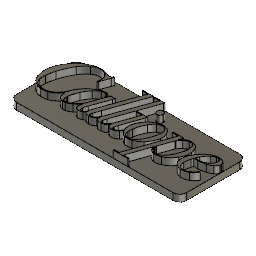
Calliope_Logo (Autodesk Fusion 360 design; units mm, degrees)
Autodesk Fusion 360 part; units mm, degrees
note: some values were not read from the file. Chosen so that the rebuilt part matches the saved one: which pieces of a blend or face edit are solid. Set by a fixed rule: which sketch regions a step uses.
(part 1 of 3)
sketch "Sketch3" plane through (0, 0, 0) normal (0, 0, 1) x (1, 0, 0)
  line L0 (156.0195, -23.5976) -> (156.0195, -61.341)
  line L1 (156.0195, -61.341) -> (108.4773, -61.341)
  spline S0 degree 3 poles (108.4773, -61.341) (108.5491, -61.0596) (108.6209, -60.7783) (108.7043, -60.4516) knots 0 0 0 0 1 1 1 1
  line L2 (108.7043, -60.4516) -> (103.7692, -60.4516)
  spline S1 degree 3 poles (103.7692, -60.4516) (106.1753, -53.6131) (108.5658, -46.8189) (110.9796, -39.9584) knots 0 0 0 0 1 1 1 1
  spline S2 degree 3 poles (110.9796, -39.9584) (111.1778, -40.6135) (111.3001, -41.1945) (111.5257, -41.7321) knots 0 0 0 0 1 1 1 1
  spline S3 degree 3 poles (111.5257, -41.7321) (112.4488, -43.9326) (114.0522, -45.3171) (116.4762, -45.532) knots 0 0 0 0 1 1 1 1
  spline S4 degree 3 poles (116.4762, -45.532) (118.5105, -45.7123) (120.4877, -45.3426) (122.343, -44.485) knots 0 0 0 0 1 1 1 1
  spline S5 degree 3 poles (122.343, -44.485) (125.9058, -42.8382) (128.6456, -40.264) (130.6312, -36.8985) knots 0 0 0 0 1 1 1 1
  spline S6 degree 3 poles (130.6312, -36.8985) (132.3382, -34.0054) (133.3231, -30.9198) (132.9158, -27.5036) knots 0 0 0 0 1 1 1 1
  spline S7 degree 3 poles (132.9158, -27.5036) (132.7164, -25.831) (132.2982, -24.2283) (131.4403, -22.7614) knots 0 0 0 0 1 1 1 1
  spline S8 degree 3 poles (131.4403, -22.7614) (129.2488, -19.0142) (125.0975, -18.1221) (121.9017, -19.2309) knots 0 0 0 0 1 1 1 1
  spline S9 degree 3 poles (121.9017, -19.2309) (119.7817, -19.9664) (118.1223, -21.3511) (116.8137, -23.1628) knots 0 0 0 0 1 1 1 1
  spline S10 degree 3 poles (116.8137, -23.1628) (116.7552, -23.2438) (116.6934, -23.3224) (116.6331, -23.4021) knots 0 0 0 0 1 1 1 1
  line L3 (116.6331, -23.4021) -> (116.5718, -23.3725)
  spline S11 degree 3 poles (116.5718, -23.3725) (116.9751, -22.1176) (117.3783, -20.8626) (117.794, -19.5691) knots 0 0 0 0 1 1 1 1
  line L4 (117.794, -19.5691) -> (117.39, -19.5691)
  spline S12 degree 3 poles (117.39, -19.5691) (116.1524, -19.5691) (114.9147, -19.5691) (113.677, -19.5691) knots 0 0 0 0 1 1 1 1
  spline S13 degree 3 poles (113.677, -19.5691) (112.0374, -19.5691) (110.3977, -19.567) (108.7581, -19.5739) knots 0 0 0 0 1 1 1 1
  spline S14 degree 3 poles (108.7581, -19.5739) (108.6477, -19.5743) (108.4711, -19.6131) (108.4397, -19.6844) knots 0 0 0 0 1 1 1 1
  spline S15 degree 3 poles (108.4397, -19.6844) (108.3413, -19.9076) (108.2979, -20.1549) (108.2252, -20.4221) knots 0 0 0 0 1 1 1 1
  line L5 (108.2252, -20.4221) -> (113.6878, -20.4221)
  spline S16 degree 3 poles (113.6878, -20.4221) (113.6473, -20.5473) (113.6177, -20.6465) (113.5834, -20.7441) knots 0 0 0 0 1 1 1 1
  spline S17 degree 3 poles (113.5834, -20.7441) (108.9605, -33.8922) (104.3365, -47.04) (99.7194, -60.1902) knots 0 0 0 0 1 1 1 1
  spline S18 degree 3 poles (99.7194, -60.1902) (99.6414, -60.4125) (99.533, -60.4699) (99.3115, -60.4681) knots 0 0 0 0 1 1 1 1
  spline S19 degree 3 poles (99.3115, -60.4681) (98.0845, -60.4581) (96.8573, -60.46) (95.6303, -60.4696) knots 0 0 0 0 1 1 1 1
  spline S20 degree 3 poles (95.6303, -60.4696) (95.5302, -60.4704) (95.3717, -60.5363) (95.342, -60.6118) knots 0 0 0 0 1 1 1 1
  spline S21 degree 3 poles (95.342, -60.6118) (95.2508, -60.8445) (95.2089, -61.0965) (95.1478, -61.341) knots 0 0 0 0 1 1 1 1
  line L6 (95.1478, -61.341) -> (0, -61.341)
  line L7 (0, -61.341) -> (0, 0)
  spline S22 degree 3 poles (0, 0) (52.0065, 0) (104.013, 0) (156.0195, 0) knots 0 0 0 0 1 1 1 1
  line L8 (156.0195, 0) -> (156.0195, -22.8998)
  spline S23 degree 3 poles (156.0195, -22.8998) (156.0019, -22.8646) (155.9715, -22.8305) (155.9685, -22.7942) knots 0 0 0 0 1 1 1 1
  spline S24 degree 3 poles (155.9685, -22.7942) (155.8892, -21.8192) (155.4189, -21.052) (154.6851, -20.4397) knots 0 0 0 0 1 1 1 1
  spline S25 degree 3 poles (154.6851, -20.4397) (153.4053, -19.3719) (151.8701, -18.9809) (150.2562, -18.8437) knots 0 0 0 0 1 1 1 1
  spline S26 degree 3 poles (150.2562, -18.8437) (147.8053, -18.6354) (145.5366, -19.2454) (143.4312, -20.4739) knots 0 0 0 0 1 1 1 1
  spline S27 degree 3 poles (143.4312, -20.4739) (139.1005, -23.0008) (136.0205, -26.6341) (134.0532, -31.2182) knots 0 0 0 0 1 1 1 1
  spline S28 degree 3 poles (134.0532, -31.2182) (133.1018, -33.4352) (132.6126, -35.7441) (132.9818, -38.1701) knots 0 0 0 0 1 1 1 1
  spline S29 degree 3 poles (132.9818, -38.1701) (133.2638, -40.0236) (133.9884, -41.6782) (135.3221, -43.0231) knots 0 0 0 0 1 1 1 1
  spline S30 degree 3 poles (135.3221, -43.0231) (136.8021, -44.5156) (138.6131, -45.3113) (140.7013, -45.5057) knots 0 0 0 0 1 1 1 1
  spline S31 degree 3 poles (140.7013, -45.5057) (143.1519, -45.7339) (145.4639, -45.3818) (147.6206, -44.0951) knots 0 0 0 0 1 1 1 1
  spline S32 degree 3 poles (147.6206, -44.0951) (149.696, -42.8569) (151.1962, -41.1095) (152.41, -39.0493) knots 0 0 0 0 1 1 1 1
  spline S33 degree 3 poles (152.41, -39.0493) (152.1937, -38.9254) (151.9691, -38.7968) (151.7296, -38.6596) knots 0 0 0 0 1 1 1 1
  spline S34 degree 3 poles (151.7296, -38.6596) (151.52, -38.9343) (151.3182, -39.1785) (151.1384, -39.4379) knots 0 0 0 0 1 1 1 1
  spline S35 degree 3 poles (151.1384, -39.4379) (150.286, -40.6676) (149.3449, -41.8167) (148.1741, -42.7628) knots 0 0 0 0 1 1 1 1
  spline S36 degree 3 poles (148.1741, -42.7628) (146.3193, -44.2615) (144.246, -45.0682) (141.8277, -44.718) knots 0 0 0 0 1 1 1 1
  spline S37 degree 3 poles (141.8277, -44.718) (139.955, -44.4468) (138.4938, -43.5447) (137.642, -41.8068) knots 0 0 0 0 1 1 1 1
  spline S38 degree 3 poles (137.642, -41.8068) (137.1687, -40.8411) (137.0345, -39.7935) (137.0087, -38.7285) knots 0 0 0 0 1 1 1 1
  spline S39 degree 3 poles (137.0087, -38.7285) (136.9596, -36.7106) (137.328, -34.757) (137.9094, -32.836) knots 0 0 0 0 1 1 1 1
  spline S40 degree 3 poles (137.9094, -32.836) (138.1099, -32.1735) (138.3185, -31.5134) (138.503, -30.9178) knots 0 0 0 0 1 1 1 1
  spline S41 degree 3 poles (138.503, -30.9178) (139.7894, -30.9729) (141.0146, -31.0989) (142.2347, -31.0619) knots 0 0 0 0 1 1 1 1
  spline S42 degree 3 poles (142.2347, -31.0619) (144.493, -30.9934) (146.7045, -30.5779) (148.8648, -29.9105) knots 0 0 0 0 1 1 1 1
  spline S43 degree 3 poles (148.8648, -29.9105) (150.5076, -29.403) (152.0871, -28.7496) (153.4759, -27.7167) knots 0 0 0 0 1 1 1 1
  spline S44 degree 3 poles (153.4759, -27.7167) (154.6089, -26.874) (155.5238, -25.8533) (155.8582, -24.4251) knots 0 0 0 0 1 1 1 1
  spline S45 degree 3 poles (155.8582, -24.4251) (155.9223, -24.1517) (155.9663, -23.8735) (156.0195, -23.5976) knots 0 0 0 0 1 1 1 1
  spline S46 degree 3 poles (50.0849, -22.4452) (50.0619, -22.439) (50.0388, -22.4327) (50.0158, -22.4265) knots 0 0 0 0 1 1 1 1
  spline S47 degree 3 poles (50.0158, -22.4265) (50.0064, -22.3974) (49.9927, -22.3689) (49.9884, -22.3392) knots 0 0 0 0 1 1 1 1
  spline S48 degree 3 poles (49.9884, -22.3392) (49.9779, -22.2661) (49.9693, -22.1925) (49.9641, -22.1189) knots 0 0 0 0 1 1 1 1
  spline S49 degree 3 poles (49.9641, -22.1189) (49.8984, -21.1818) (49.4912, -20.4209) (48.7702, -19.8267) knots 0 0 0 0 1 1 1 1
  spline S50 degree 3 poles (48.7702, -19.8267) (47.7681, -19.0007) (46.5961, -18.7389) (45.3289, -18.8182) knots 0 0 0 0 1 1 1 1
  spline S51 degree 3 poles (45.3289, -18.8182) (43.9034, -18.9073) (42.5718, -19.3541) (41.2975, -19.9603) knots 0 0 0 0 1 1 1 1
  spline S52 degree 3 poles (41.2975, -19.9603) (37.4617, -21.785) (34.2471, -24.4068) (31.5841, -27.6967) knots 0 0 0 0 1 1 1 1
  spline S53 degree 3 poles (31.5841, -27.6967) (29.8681, -29.8167) (28.5608, -32.172) (27.7761, -34.8009) knots 0 0 0 0 1 1 1 1
  spline S54 degree 3 poles (27.7761, -34.8009) (27.6548, -35.2071) (27.6013, -35.6146) (27.2979, -35.9909) knots 0 0 0 0 1 1 1 1
  spline S55 degree 3 poles (27.2979, -35.9909) (26.7981, -36.6105) (26.4452, -37.3469) (26.0145, -38.024) knots 0 0 0 0 1 1 1 1
  spline S56 degree 3 poles (26.0145, -38.024) (24.3785, -40.5957) (22.1935, -42.5594) (19.4153, -43.8207) knots 0 0 0 0 1 1 1 1
  spline S57 degree 3 poles (19.4153, -43.8207) (16.336, -45.2186) (13.1649, -45.1705) (10.0109, -44.1478) knots 0 0 0 0 1 1 1 1
  spline S58 degree 3 poles (10.0109, -44.1478) (7.3021, -43.2695) (5.6053, -41.3794) (4.9304, -38.5933) knots 0 0 0 0 1 1 1 1
  spline S59 degree 3 poles (4.9304, -38.5933) (4.4781, -36.726) (4.5193, -34.842) (4.7229, -32.9543) knots 0 0 0 0 1 1 1 1
  spline S60 degree 3 poles (4.7229, -32.9543) (5.0136, -30.2599) (5.5761, -27.6183) (6.3535, -25.0241) knots 0 0 0 0 1 1 1 1
  spline S61 degree 3 poles (6.3535, -25.0241) (7.7161, -20.4766) (9.4965, -16.1067) (12.0128, -12.064) knots 0 0 0 0 1 1 1 1
  spline S62 degree 3 poles (12.0128, -12.064) (13.6498, -9.4342) (15.5983, -7.0752) (18.1065, -5.2075) knots 0 0 0 0 1 1 1 1
  spline S63 degree 3 poles (18.1065, -5.2075) (21.6115, -2.5974) (25.4024, -2.3618) (29.3636, -3.8873) knots 0 0 0 0 1 1 1 1
  spline S64 degree 3 poles (29.3636, -3.8873) (31.4072, -4.6744) (32.7504, -6.1919) (33.298, -8.3429) knots 0 0 0 0 1 1 1 1
  spline S65 degree 3 poles (33.298, -8.3429) (33.6344, -9.6642) (33.5355, -11.0084) (33.4161, -12.3468) knots 0 0 0 0 1 1 1 1
  spline S66 degree 3 poles (33.4161, -12.3468) (33.3593, -12.9843) (33.2661, -13.6185) (33.1895, -14.2539) knots 0 0 0 0 1 1 1 1
  spline S67 degree 3 poles (33.1895, -14.2539) (33.924, -14.3486) (33.9218, -14.3478) (34.1497, -13.71) knots 0 0 0 0 1 1 1 1
  spline S68 degree 3 poles (34.1497, -13.71) (35.1509, -10.908) (36.1535, -8.1065) (37.1555, -5.3048) knots 0 0 0 0 1 1 1 1
  spline S69 degree 3 poles (37.1555, -5.3048) (37.4387, -4.513) (37.7215, -3.721) (38.014, -2.9026) knots 0 0 0 0 1 1 1 1
  spline S70 degree 3 poles (38.014, -2.9026) (37.8301, -2.8616) (37.6735, -2.8421) (37.5281, -2.7909) knots 0 0 0 0 1 1 1 1
  spline S71 degree 3 poles (37.5281, -2.7909) (37.2322, -2.6868) (37.0752, -2.7732) (36.9084, -3.0554) knots 0 0 0 0 1 1 1 1
  spline S72 degree 3 poles (36.9084, -3.0554) (36.3629, -3.9783) (35.5622, -4.5251) (34.4509, -4.4166) knots 0 0 0 0 1 1 1 1
  spline S73 degree 3 poles (34.4509, -4.4166) (33.9099, -4.3637) (33.3658, -4.2376) (32.8488, -4.0667) knots 0 0 0 0 1 1 1 1
  spline S74 degree 3 poles (32.8488, -4.0667) (31.9676, -3.7753) (31.1102, -3.4127) (30.2365, -3.0973) knots 0 0 0 0 1 1 1 1
  spline S75 degree 3 poles (30.2365, -3.0973) (27.7778, -2.2096) (25.2539, -1.9088) (22.6573, -2.2749) knots 0 0 0 0 1 1 1 1
  spline S76 degree 3 poles (22.6573, -2.2749) (20.7362, -2.5458) (18.9175, -3.1537) (17.1711, -3.9759) knots 0 0 0 0 1 1 1 1
  spline S77 degree 3 poles (17.1711, -3.9759) (11.8716, -6.4708) (7.6391, -10.2081) (4.4487, -15.0988) knots 0 0 0 0 1 1 1 1
  spline S78 degree 3 poles (4.4487, -15.0988) (1.4603, -19.6798) (-0.1988, -24.667) (0.1153, -30.2088) knots 0 0 0 0 1 1 1 1
  spline S79 degree 3 poles (0.1153, -30.2088) (0.2462, -32.5189) (0.589, -34.789) (1.4018, -36.9651) knots 0 0 0 0 1 1 1 1
  spline S80 degree 3 poles (1.4018, -36.9651) (2.7269, -40.5128) (5.07, -43.1219) (8.5869, -44.6156) knots 0 0 0 0 1 1 1 1
  spline S81 degree 3 poles (8.5869, -44.6156) (9.982, -45.2081) (11.4556, -45.483) (12.9615, -45.5794) knots 0 0 0 0 1 1 1 1
  spline S82 degree 3 poles (12.9615, -45.5794) (14.9147, -45.7043) (16.8656, -45.6654) (18.7272, -44.9928) knots 0 0 0 0 1 1 1 1
  spline S83 degree 3 poles (18.7272, -44.9928) (22.1612, -43.7524) (24.8613, -41.5667) (26.8476, -38.5034) knots 0 0 0 0 1 1 1 1
  spline S84 degree 3 poles (26.8476, -38.5034) (26.988, -38.287) (27.118, -38.0638) (27.2529, -37.8437) knots 0 0 0 0 1 1 1 1
  spline S85 degree 3 poles (27.2529, -37.8437) (27.3252, -37.9926) (27.3127, -38.1253) (27.3273, -38.2549) knots 0 0 0 0 1 1 1 1
  spline S86 degree 3 poles (27.3273, -38.2549) (27.4213, -39.0926) (27.4431, -39.948) (27.6348, -40.7633) knots 0 0 0 0 1 1 1 1
  spline S87 degree 3 poles (27.6348, -40.7633) (28.0824, -42.6659) (29.1177, -44.1579) (30.9434, -45.0023) knots 0 0 0 0 1 1 1 1
  spline S88 degree 3 poles (30.9434, -45.0023) (32.3176, -45.6378) (33.7642, -45.6821) (35.2298, -45.4504) knots 0 0 0 0 1 1 1 1
  spline S89 degree 3 poles (35.2298, -45.4504) (37.0632, -45.1607) (38.6343, -44.293) (40.0946, -43.1941) knots 0 0 0 0 1 1 1 1
  spline S90 degree 3 poles (40.0946, -43.1941) (41.6556, -42.0196) (42.8844, -40.5225) (44.1283, -39.0402) knots 0 0 0 0 1 1 1 1
  spline S91 degree 3 poles (44.1283, -39.0402) (44.2114, -38.9412) (44.2975, -38.8447) (44.3823, -38.747) knots 0 0 0 0 1 1 1 1
  spline S92 degree 3 poles (44.3823, -38.747) (44.4123, -38.9053) (44.3802, -39.0239) (44.3478, -39.1425) knots 0 0 0 0 1 1 1 1
  spline S93 degree 3 poles (44.3478, -39.1425) (44.0412, -40.2656) (43.7805, -41.3953) (43.8608, -42.5731) knots 0 0 0 0 1 1 1 1
  spline S94 degree 3 poles (43.8608, -42.5731) (43.9596, -44.0239) (44.7538, -45.0434) (46.147, -45.3786) knots 0 0 0 0 1 1 1 1
  spline S95 degree 3 poles (46.147, -45.3786) (47.775, -45.7703) (49.3655, -45.6409) (50.8342, -44.773) knots 0 0 0 0 1 1 1 1
  spline S96 degree 3 poles (50.8342, -44.773) (51.4483, -44.4101) (52.0194, -43.9749) (52.6073, -43.5745) knots 0 0 0 0 1 1 1 1
  spline S97 degree 3 poles (52.6073, -43.5745) (53.0764, -44.5495) (53.5786, -45.0228) (54.6679, -45.2941) knots 0 0 0 0 1 1 1 1
  spline S98 degree 3 poles (54.6679, -45.2941) (55.3375, -45.4608) (56.041, -45.5543) (56.731, -45.5649) knots 0 0 0 0 1 1 1 1
  spline S99 degree 3 poles (56.731, -45.5649) (58.821, -45.5971) (60.4965, -44.6726) (61.8903, -43.1798) knots 0 0 0 0 1 1 1 1
  spline S100 degree 3 poles (61.8903, -43.1798) (62.2327, -42.813) (62.5336, -42.4076) (62.8925, -41.9728) knots 0 0 0 0 1 1 1 1
  spline S101 degree 3 poles (62.8925, -41.9728) (62.8925, -42.1445) (62.8903, -42.2662) (62.8928, -42.3877) knots 0 0 0 0 1 1 1 1
  spline S102 degree 3 poles (62.8928, -42.3877) (62.9231, -43.8262) (63.5858, -44.7511) (64.9382, -45.2356) knots 0 0 0 0 1 1 1 1
  spline S103 degree 3 poles (64.9382, -45.2356) (65.967, -45.6042) (67.0307, -45.6375) (68.0997, -45.5148) knots 0 0 0 0 1 1 1 1
  spline S104 degree 3 poles (68.0997, -45.5148) (69.8832, -45.31) (71.2784, -44.3806) (72.4656, -43.096) knots 0 0 0 0 1 1 1 1
  spline S105 degree 3 poles (72.4656, -43.096) (72.7758, -42.7603) (73.0458, -42.3875) (73.3767, -41.9795) knots 0 0 0 0 1 1 1 1
  spline S106 degree 3 poles (73.3767, -41.9795) (73.3767, -42.1348) (73.3743, -42.2262) (73.3771, -42.3173) knots 0 0 0 0 1 1 1 1
  spline S107 degree 3 poles (73.3771, -42.3173) (73.4271, -43.9443) (74.2035, -44.9618) (75.7898, -45.3455) knots 0 0 0 0 1 1 1 1
  spline S108 degree 3 poles (75.7898, -45.3455) (78.4926, -45.9992) (80.8441, -45.3252) (82.7546, -43.3024) knots 0 0 0 0 1 1 1 1
  spline S109 degree 3 poles (82.7546, -43.3024) (83.3917, -42.6279) (83.8997, -41.8316) (84.4745, -41.0809) knots 0 0 0 0 1 1 1 1
  spline S110 degree 3 poles (84.4745, -41.0809) (84.4258, -41.054) (84.4504, -41.0594) (84.4605, -41.0746) knots 0 0 0 0 1 1 1 1
  spline S111 degree 3 poles (84.4605, -41.0746) (84.5133, -41.1535) (84.5617, -41.2351) (84.6127, -41.3152) knots 0 0 0 0 1 1 1 1
  spline S112 degree 3 poles (84.6127, -41.3152) (85.7145, -43.047) (87.2073, -44.3196) (89.1334, -45.0354) knots 0 0 0 0 1 1 1 1
  spline S113 degree 3 poles (89.1334, -45.0354) (91.3614, -45.8636) (93.5987, -45.7048) (95.8081, -44.9373) knots 0 0 0 0 1 1 1 1
  spline S114 degree 3 poles (95.8081, -44.9373) (98.3827, -44.0429) (100.6013, -42.5754) (102.4686, -40.6044) knots 0 0 0 0 1 1 1 1
  spline S115 degree 3 poles (102.4686, -40.6044) (105.1593, -37.7643) (107.0753, -34.5158) (107.5538, -30.5511) knots 0 0 0 0 1 1 1 1
  spline S116 degree 3 poles (107.5538, -30.5511) (107.8486, -28.1077) (107.5188, -25.7593) (106.3628, -23.5722) knots 0 0 0 0 1 1 1 1
  spline S117 degree 3 poles (106.3628, -23.5722) (105.1687, -21.313) (103.3851, -19.714) (100.8692, -19.0689) knots 0 0 0 0 1 1 1 1
  spline S118 degree 3 poles (100.8692, -19.0689) (98.8651, -18.5551) (96.8679, -18.7479) (94.9427, -19.4482) knots 0 0 0 0 1 1 1 1
  spline S119 degree 3 poles (94.9427, -19.4482) (89.5691, -21.4031) (85.9017, -25.1273) (83.9323, -30.4535) knots 0 0 0 0 1 1 1 1
  spline S120 degree 3 poles (83.9323, -30.4535) (82.7766, -33.5787) (82.6174, -36.7855) (83.9032, -39.9585) knots 0 0 0 0 1 1 1 1
  spline S121 degree 3 poles (83.9032, -39.9585) (83.9365, -40.0409) (83.9344, -40.169) (83.893, -40.2456) knots 0 0 0 0 1 1 1 1
  spline S122 degree 3 poles (83.893, -40.2456) (83.0471, -41.8113) (81.9568, -43.1756) (80.4699, -44.1743) knots 0 0 0 0 1 1 1 1
  spline S123 degree 3 poles (80.4699, -44.1743) (80.0606, -44.4492) (79.5647, -44.644) (79.081, -44.7494) knots 0 0 0 0 1 1 1 1
  spline S124 degree 3 poles (79.081, -44.7494) (78.0389, -44.9766) (77.2211, -44.4149) (77.0795, -43.4251) knots 0 0 0 0 1 1 1 1
  spline S125 degree 3 poles (77.0795, -43.4251) (77.0352, -43.1161) (77.0232, -42.7789) (77.0991, -42.4806) knots 0 0 0 0 1 1 1 1
  spline S126 degree 3 poles (77.0991, -42.4806) (77.3431, -41.5214) (77.5918, -40.5594) (77.9153, -39.625) knots 0 0 0 0 1 1 1 1
  spline S127 degree 3 poles (77.9153, -39.625) (80.0449, -33.4733) (82.1947, -27.3287) (84.3372, -21.1815) knots 0 0 0 0 1 1 1 1
  spline S128 degree 3 poles (84.3372, -21.1815) (84.5194, -20.6587) (84.6969, -20.1342) (84.8909, -19.5691) knots 0 0 0 0 1 1 1 1
  line L9 (84.8909, -19.5691) -> (84.4958, -19.5691)
  spline S129 degree 3 poles (84.4958, -19.5691) (83.6071, -19.5691) (82.7185, -19.5691) (81.8299, -19.5691) knots 0 0 0 0 1 1 1 1
  spline S130 degree 3 poles (81.8299, -19.5691) (79.82, -19.5691) (77.81, -19.5675) (75.8, -19.5737) knots 0 0 0 0 1 1 1 1
  spline S131 degree 3 poles (75.8, -19.5737) (75.6902, -19.574) (75.5152, -19.6102) (75.4831, -19.6808) knots 0 0 0 0 1 1 1 1
  spline S132 degree 3 poles (75.4831, -19.6808) (75.3826, -19.9022) (75.336, -20.148) (75.2552, -20.4306) knots 0 0 0 0 1 1 1 1
  line L10 (75.2552, -20.4306) -> (80.4962, -20.4306)
  spline S133 degree 3 poles (80.4962, -20.4306) (80.4479, -20.5681) (80.4134, -20.6665) (80.3788, -20.7648) knots 0 0 0 0 1 1 1 1
  spline S134 degree 3 poles (80.3788, -20.7648) (78.5197, -26.0499) (76.6624, -31.3356) (74.7999, -36.6195) knots 0 0 0 0 1 1 1 1
  spline S135 degree 3 poles (74.7999, -36.6195) (74.4293, -37.6709) (74.1085, -38.7475) (73.6419, -39.7556) knots 0 0 0 0 1 1 1 1
  spline S136 degree 3 poles (73.6419, -39.7556) (72.8455, -41.4761) (71.6905, -42.9385) (70.1463, -44.0705) knots 0 0 0 0 1 1 1 1
  spline S137 degree 3 poles (70.1463, -44.0705) (69.6796, -44.4126) (69.1749, -44.6659) (68.5994, -44.764) knots 0 0 0 0 1 1 1 1
  spline S138 degree 3 poles (68.5994, -44.764) (67.3793, -44.9721) (66.5417, -44.2641) (66.5563, -43.0267) knots 0 0 0 0 1 1 1 1
  spline S139 degree 3 poles (66.5563, -43.0267) (66.5593, -42.7745) (66.5643, -42.5124) (66.6319, -42.2727) knots 0 0 0 0 1 1 1 1
  spline S140 degree 3 poles (66.6319, -42.2727) (66.8922, -41.3499) (67.1403, -40.4209) (67.4606, -39.5181) knots 0 0 0 0 1 1 1 1
  spline S141 degree 3 poles (67.4606, -39.5181) (71.9791, -26.78) (76.5089, -14.0458) (81.0355, -1.3105) knots 0 0 0 0 1 1 1 1
  spline S142 degree 3 poles (81.0355, -1.3105) (81.1791, -0.9064) (81.3172, -0.5003) (81.469, -0.0634) knots 0 0 0 0 1 1 1 1
  line L11 (81.469, -0.0634) -> (81.0443, -0.0634)
  spline S143 degree 3 poles (81.0443, -0.0634) (78.2938, -0.0634) (75.5433, -0.0634) (72.7928, -0.0634) knots 0 0 0 0 1 1 1 1
  spline S144 degree 2 poles (72.7928, -0.0634) (72.0388, -0.0634) (71.87, -0.8059) knots 0 0 0 1 1 1
  spline S145 degree 3 poles (71.87, -0.8059) (71.8656, -0.8253) (71.8729, -0.8474) (71.8772, -0.8969) knots 0 0 0 0 1 1 1 1
  line L12 (71.8772, -0.8969) -> (77.0797, -0.8969)
  spline S146 degree 3 poles (77.0797, -0.8969) (77.0261, -1.0528) (76.9874, -1.1697) (76.946, -1.2857) knots 0 0 0 0 1 1 1 1
  spline S147 degree 3 poles (76.946, -1.2857) (72.7448, -13.0394) (68.5443, -24.7933) (64.3408, -36.5461) knots 0 0 0 0 1 1 1 1
  spline S148 degree 3 poles (64.3408, -36.5461) (63.951, -37.6361) (63.6149, -38.7533) (63.1258, -39.7979) knots 0 0 0 0 1 1 1 1
  spline S149 degree 3 poles (63.1258, -39.7979) (62.2985, -41.5649) (61.1119, -43.0774) (59.4732, -44.176) knots 0 0 0 0 1 1 1 1
  spline S150 degree 3 poles (59.4732, -44.176) (59.0639, -44.4504) (58.5683, -44.6503) (58.0846, -44.749) knots 0 0 0 0 1 1 1 1
  spline S151 degree 3 poles (58.0846, -44.749) (56.8852, -44.9938) (56.0307, -44.2662) (56.0713, -43.0432) knots 0 0 0 0 1 1 1 1
  spline S152 degree 3 poles (56.0713, -43.0432) (56.0896, -42.4913) (56.1806, -41.9219) (56.3538, -41.3986) knots 0 0 0 0 1 1 1 1
  spline S153 degree 3 poles (56.3538, -41.3986) (57.0233, -39.3758) (57.7269, -37.364) (58.4397, -35.3559) knots 0 0 0 0 1 1 1 1
  spline S154 degree 3 poles (58.4397, -35.3559) (62.5801, -23.6925) (66.7268, -12.0314) (70.8707, -0.3694) knots 0 0 0 0 1 1 1 1
  spline S155 degree 3 poles (70.8707, -0.3694) (70.9037, -0.2765) (70.9286, -0.1807) (70.961, -0.0737) knots 0 0 0 0 1 1 1 1
  line L13 (70.961, -0.0737) -> (61.5817, -0.0737)
  spline S156 degree 3 poles (61.5817, -0.0737) (61.5071, -0.3392) (61.434, -0.5992) (61.3495, -0.8998) knots 0 0 0 0 1 1 1 1
  line L14 (61.3495, -0.8998) -> (66.5754, -0.8998)
  spline S157 degree 3 poles (66.5754, -0.8998) (66.5356, -1.0258) (66.5105, -1.1153) (66.4793, -1.2026) knots 0 0 0 0 1 1 1 1
  spline S158 degree 3 poles (66.4793, -1.2026) (63.3253, -10.0253) (60.1699, -18.8474) (57.0169, -27.6704) knots 0 0 0 0 1 1 1 1
  spline S159 degree 3 poles (57.0169, -27.6704) (55.7387, -31.2473) (54.4525, -34.8214) (53.1977, -38.4066) knots 0 0 0 0 1 1 1 1
  spline S160 degree 3 poles (53.1977, -38.4066) (52.7378, -39.7205) (52.2958, -41.0495) (52.3874, -42.4803) knots 0 0 0 0 1 1 1 1
  spline S161 degree 3 poles (52.3874, -42.4803) (52.3929, -42.5673) (52.3208, -42.6844) (52.2494, -42.7473) knots 0 0 0 0 1 1 1 1
  spline S162 degree 3 poles (52.2494, -42.7473) (51.8299, -43.117) (51.4215, -43.505) (50.9682, -43.8296) knots 0 0 0 0 1 1 1 1
  spline S163 degree 3 poles (50.9682, -43.8296) (50.2819, -44.3211) (49.495, -44.5041) (48.6533, -44.4098) knots 0 0 0 0 1 1 1 1
  spline S164 degree 3 poles (48.6533, -44.4098) (48.0159, -44.3384) (47.5969, -43.9415) (47.5472, -43.3015) knots 0 0 0 0 1 1 1 1
  spline S165 degree 3 poles (47.5472, -43.3015) (47.5124, -42.8522) (47.5238, -42.3918) (47.5794, -41.9443) knots 0 0 0 0 1 1 1 1
  spline S166 degree 3 poles (47.5794, -41.9443) (47.7533, -40.5433) (48.1881, -39.2037) (48.6587, -37.8828) knots 0 0 0 0 1 1 1 1
  spline S167 degree 3 poles (48.6587, -37.8828) (50.6099, -32.4064) (52.5864, -26.939) (54.5533, -21.4682) knots 0 0 0 0 1 1 1 1
  spline S168 degree 3 poles (54.5533, -21.4682) (54.7762, -20.8484) (54.9976, -20.2281) (55.2275, -19.5862) knots 0 0 0 0 1 1 1 1
  spline S169 degree 3 poles (55.2275, -19.5862) (55.1098, -19.5785) (55.0374, -19.5698) (54.965, -19.5698) knots 0 0 0 0 1 1 1 1
  spline S170 degree 3 poles (54.965, -19.5698) (53.7273, -19.5691) (52.4896, -19.5659) (51.252, -19.5784) knots 0 0 0 0 1 1 1 1
  spline S171 degree 3 poles (51.252, -19.5784) (51.1737, -19.5792) (51.0605, -19.6886) (51.0256, -19.7731) knots 0 0 0 0 1 1 1 1
  spline S172 degree 3 poles (51.0256, -19.7731) (50.9049, -20.0653) (50.8124, -20.369) (50.7079, -20.6679) knots 0 0 0 0 1 1 1 1
  spline S173 degree 3 poles (50.7079, -20.6679) (50.5007, -21.2605) (50.2927, -21.8528) (50.085, -22.4452) knots 0 0 0 0 1 1 1 1
  line L15 (50.085, -22.4452) -> (50.0849, -22.4452)
  spline S174 degree 3 poles (84.1667, -10.1913) (84.1605, -11.7915) (85.3374, -12.9908) (86.9258, -13.0029) knots 0 0 0 0 1 1 1 1
  spline S175 degree 3 poles (86.9258, -13.0029) (88.5136, -13.0149) (89.7183, -11.8206) (89.7211, -10.2316) knots 0 0 0 0 1 1 1 1
  spline S176 degree 3 poles (89.7211, -10.2316) (89.7239, -8.6369) (88.5314, -7.4321) (86.9503, -7.4324) knots 0 0 0 0 1 1 1 1
  spline S177 degree 3 poles (86.9503, -7.4324) (85.3768, -7.4326) (84.1729, -8.6259) (84.1667, -10.1913) knots 0 0 0 0 1 1 1 1
  spline S178 degree 3 poles (95.1478, -61.341) (95.2089, -61.0965) (95.2508, -60.8445) (95.342, -60.6118) knots 0 0 0 0 1 1 1 1
  spline S179 degree 3 poles (95.342, -60.6118) (95.3717, -60.5363) (95.5302, -60.4704) (95.6303, -60.4696) knots 0 0 0 0 1 1 1 1
  spline S180 degree 3 poles (95.6303, -60.4696) (96.8573, -60.46) (98.0845, -60.4581) (99.3115, -60.4681) knots 0 0 0 0 1 1 1 1
  spline S181 degree 3 poles (99.3115, -60.4681) (99.5329, -60.4699) (99.6414, -60.4125) (99.7194, -60.1902) knots 0 0 0 0 1 1 1 1
  spline S182 degree 3 poles (99.7194, -60.1902) (104.3365, -47.04) (108.9605, -33.8922) (113.5834, -20.7441) knots 0 0 0 0 1 1 1 1
  spline S183 degree 3 poles (113.5834, -20.7441) (113.6177, -20.6465) (113.6473, -20.5473) (113.6878, -20.4221) knots 0 0 0 0 1 1 1 1
  line L16 (113.6878, -20.4221) -> (108.2252, -20.4221)
  spline S184 degree 3 poles (108.2252, -20.4221) (108.2979, -20.1549) (108.3413, -19.9076) (108.4397, -19.6844) knots 0 0 0 0 1 1 1 1
  spline S185 degree 3 poles (108.4397, -19.6844) (108.4711, -19.6131) (108.6477, -19.5743) (108.7581, -19.5739) knots 0 0 0 0 1 1 1 1
  spline S186 degree 3 poles (108.7581, -19.5739) (110.3977, -19.567) (112.0374, -19.5691) (113.677, -19.5691) knots 0 0 0 0 1 1 1 1
  spline S187 degree 3 poles (113.677, -19.5691) (114.9147, -19.5691) (116.1524, -19.5691) (117.39, -19.5691) knots 0 0 0 0 1 1 1 1
  line L17 (117.39, -19.5691) -> (117.794, -19.5691)
  spline S188 degree 3 poles (117.794, -19.5691) (117.3783, -20.8626) (116.9751, -22.1176) (116.5718, -23.3725) knots 0 0 0 0 1 1 1 1
  line L18 (116.5718, -23.3725) -> (116.6331, -23.4021)
  spline S189 degree 3 poles (116.6331, -23.4021) (116.6934, -23.3224) (116.7552, -23.2438) (116.8137, -23.1628) knots 0 0 0 0 1 1 1 1
  spline S190 degree 3 poles (116.8137, -23.1628) (118.1223, -21.3511) (119.7817, -19.9664) (121.9017, -19.2309) knots 0 0 0 0 1 1 1 1
  spline S191 degree 3 poles (121.9017, -19.2309) (125.0975, -18.1221) (129.2488, -19.0142) (131.4403, -22.7614) knots 0 0 0 0 1 1 1 1
  spline S192 degree 3 poles (131.4403, -22.7614) (132.2982, -24.2283) (132.7164, -25.831) (132.9158, -27.5036) knots 0 0 0 0 1 1 1 1
  spline S193 degree 3 poles (132.9158, -27.5036) (133.3231, -30.9198) (132.3382, -34.0053) (130.6312, -36.8985) knots 0 0 0 0 1 1 1 1
  spline S194 degree 3 poles (130.6312, -36.8985) (128.6456, -40.264) (125.9058, -42.8382) (122.343, -44.485) knots 0 0 0 0 1 1 1 1
  spline S195 degree 3 poles (122.343, -44.485) (120.4877, -45.3426) (118.5105, -45.7123) (116.4762, -45.532) knots 0 0 0 0 1 1 1 1
  spline S196 degree 3 poles (116.4762, -45.532) (114.0521, -45.3171) (112.4488, -43.9326) (111.5257, -41.7321) knots 0 0 0 0 1 1 1 1
  spline S197 degree 3 poles (111.5257, -41.7321) (111.3001, -41.1945) (111.1778, -40.6135) (110.9796, -39.9584) knots 0 0 0 0 1 1 1 1
  spline S198 degree 3 poles (110.9796, -39.9584) (108.5658, -46.8189) (106.1753, -53.6131) (103.7692, -60.4516) knots 0 0 0 0 1 1 1 1
  line L19 (103.7692, -60.4516) -> (108.7043, -60.4516)
  spline S199 degree 3 poles (108.7043, -60.4516) (108.6209, -60.7782) (108.5491, -61.0596) (108.4773, -61.341) knots 0 0 0 0 1 1 1 1
  line L20 (108.4773, -61.341) -> (95.1478, -61.341)
  spline S200 degree 3 poles (128.8614, -26.1716) (128.8638, -24.552) (128.6621, -23.2915) (128.1613, -22.0809) knots 0 0 0 0 1 1 1 1
  spline S201 degree 3 poles (128.1613, -22.0809) (127.6838, -20.9266) (126.9085, -20.1109) (125.6676, -19.8061) knots 0 0 0 0 1 1 1 1
  spline S202 degree 3 poles (125.6676, -19.8061) (124.8028, -19.5937) (123.9276, -19.5934) (123.056, -19.7578) knots 0 0 0 0 1 1 1 1
  spline S203 degree 3 poles (123.056, -19.7578) (121.5941, -20.0336) (120.4047, -20.8235) (119.3159, -21.7871) knots 0 0 0 0 1 1 1 1
  spline S204 degree 3 poles (119.3159, -21.7871) (118.185, -22.7878) (117.2705, -23.9794) (116.3717, -25.182) knots 0 0 0 0 1 1 1 1
  spline S205 degree 3 poles (116.3717, -25.182) (116.2291, -25.3728) (116.1079, -25.5914) (116.0281, -25.8153) knots 0 0 0 0 1 1 1 1
  spline S206 degree 3 poles (116.0281, -25.8153) (114.5515, -29.9585) (113.0797, -34.1034) (111.6206, -38.2527) knots 0 0 0 0 1 1 1 1
  spline S207 degree 3 poles (111.6206, -38.2527) (111.5424, -38.4751) (111.5353, -38.7499) (111.5818, -38.983) knots 0 0 0 0 1 1 1 1
  spline S208 degree 3 poles (111.5818, -38.983) (111.687, -39.5095) (111.834, -40.0287) (111.9863, -40.5443) knots 0 0 0 0 1 1 1 1
  spline S209 degree 3 poles (111.9863, -40.5443) (112.3341, -41.7221) (112.9324, -42.7442) (113.845, -43.5861) knots 0 0 0 0 1 1 1 1
  spline S210 degree 3 poles (113.845, -43.5861) (115.4801, -45.0946) (118.0331, -45.0928) (119.806, -44.129) knots 0 0 0 0 1 1 1 1
  spline S211 degree 3 poles (119.806, -44.129) (121.3489, -43.2903) (122.5648, -42.0801) (123.61, -40.6911) knots 0 0 0 0 1 1 1 1
  spline S212 degree 3 poles (123.61, -40.6911) (125.3817, -38.3368) (126.5931, -35.6965) (127.5153, -32.9166) knots 0 0 0 0 1 1 1 1
  spline S213 degree 3 poles (127.5153, -32.9166) (128.276, -30.6235) (128.8153, -28.284) (128.8614, -26.1716) knots 0 0 0 0 1 1 1 1
  spline S214 degree 3 poles (156.0195, -23.5976) (155.9663, -23.8735) (155.9222, -24.1517) (155.8582, -24.4251) knots 0 0 0 0 1 1 1 1
  spline S215 degree 3 poles (155.8582, -24.4251) (155.5238, -25.8533) (154.6088, -26.874) (153.4759, -27.7167) knots 0 0 0 0 1 1 1 1
  spline S216 degree 3 poles (153.4759, -27.7167) (152.0871, -28.7496) (150.5076, -29.403) (148.8648, -29.9105) knots 0 0 0 0 1 1 1 1
  spline S217 degree 3 poles (148.8648, -29.9105) (146.7045, -30.5779) (144.493, -30.9934) (142.2347, -31.0619) knots 0 0 0 0 1 1 1 1
  spline S218 degree 3 poles (142.2347, -31.0619) (141.0145, -31.0989) (139.7894, -30.9729) (138.503, -30.9178) knots 0 0 0 0 1 1 1 1
  spline S219 degree 3 poles (138.503, -30.9178) (138.3184, -31.5134) (138.1099, -32.1735) (137.9094, -32.836) knots 0 0 0 0 1 1 1 1
  spline S220 degree 3 poles (137.9094, -32.836) (137.328, -34.757) (136.9596, -36.7106) (137.0087, -38.7285) knots 0 0 0 0 1 1 1 1
  spline S221 degree 3 poles (137.0087, -38.7285) (137.0345, -39.7935) (137.1687, -40.8411) (137.642, -41.8068) knots 0 0 0 0 1 1 1 1
  spline S222 degree 3 poles (137.642, -41.8068) (138.4938, -43.5447) (139.955, -44.4468) (141.8277, -44.718) knots 0 0 0 0 1 1 1 1
  spline S223 degree 3 poles (141.8277, -44.718) (144.246, -45.0682) (146.3193, -44.2615) (148.1741, -42.7628) knots 0 0 0 0 1 1 1 1
  spline S224 degree 3 poles (148.1741, -42.7628) (149.3448, -41.8167) (150.286, -40.6676) (151.1384, -39.4379) knots 0 0 0 0 1 1 1 1
  spline S225 degree 3 poles (151.1384, -39.4379) (151.3182, -39.1785) (151.52, -38.9343) (151.7296, -38.6596) knots 0 0 0 0 1 1 1 1
  spline S226 degree 3 poles (151.7296, -38.6596) (151.9691, -38.7968) (152.1937, -38.9254) (152.41, -39.0493) knots 0 0 0 0 1 1 1 1
  spline S227 degree 3 poles (152.41, -39.0493) (151.1962, -41.1095) (149.6959, -42.8569) (147.6206, -44.0951) knots 0 0 0 0 1 1 1 1
  spline S228 degree 3 poles (147.6206, -44.0951) (145.4638, -45.3818) (143.1519, -45.7339) (140.7013, -45.5057) knots 0 0 0 0 1 1 1 1
  spline S229 degree 3 poles (140.7013, -45.5057) (138.6131, -45.3113) (136.8021, -44.5156) (135.3221, -43.0231) knots 0 0 0 0 1 1 1 1
  spline S230 degree 3 poles (132.9818, -38.1701) (132.6126, -35.7441) (133.1018, -33.4352) (134.0532, -31.2182) knots 0 0 0 0 1 1 1 1
  spline S231 degree 3 poles (134.0532, -31.2182) (136.0205, -26.6341) (139.1004, -23.0008) (143.4312, -20.4739) knots 0 0 0 0 1 1 1 1
  spline S232 degree 3 poles (143.4312, -20.4739) (145.5366, -19.2454) (147.8053, -18.6354) (150.2562, -18.8437) knots 0 0 0 0 1 1 1 1
  spline S233 degree 3 poles (150.2562, -18.8437) (151.8701, -18.9809) (153.4053, -19.3719) (154.6851, -20.4397) knots 0 0 0 0 1 1 1 1
  spline S234 degree 3 poles (154.6851, -20.4397) (155.4188, -21.052) (155.8891, -21.8192) (155.9685, -22.7942) knots 0 0 0 0 1 1 1 1
  spline S235 degree 3 poles (155.9685, -22.7942) (155.9715, -22.8305) (156.0019, -22.8646) (156.0195, -22.8998) knots 0 0 0 0 1 1 1 1
  line L21 (156.0195, -22.8998) -> (156.0195, -23.5976)
  spline S236 degree 3 poles (138.7712, -30.0038) (139.2833, -30.0649) (139.7002, -30.1254) (140.1191, -30.1628) knots 0 0 0 0 1 1 1 1
  spline S237 degree 3 poles (140.1191, -30.1628) (142.2832, -30.356) (144.4026, -30.1915) (146.4395, -29.3662) knots 0 0 0 0 1 1 1 1
  spline S238 degree 3 poles (146.4395, -29.3662) (148.2949, -28.6145) (149.935, -27.569) (151.122, -25.9174) knots 0 0 0 0 1 1 1 1
  spline S239 degree 3 poles (151.122, -25.9174) (151.9809, -24.7224) (152.4727, -23.4101) (152.2726, -21.9102) knots 0 0 0 0 1 1 1 1
  spline S240 degree 3 poles (152.2726, -21.9102) (152.1161, -20.7367) (151.3327, -19.8797) (150.1687, -19.7408) knots 0 0 0 0 1 1 1 1
  spline S241 degree 3 poles (150.1687, -19.7408) (149.4761, -19.6581) (148.7512, -19.6761) (148.0608, -19.7806) knots 0 0 0 0 1 1 1 1
  spline S242 degree 3 poles (148.0608, -19.7806) (146.7386, -19.9808) (145.6448, -20.6992) (144.619, -21.5155) knots 0 0 0 0 1 1 1 1
  spline S243 degree 3 poles (144.619, -21.5155) (142.6739, -23.0631) (141.2378, -25.0227) (140.0927, -27.2034) knots 0 0 0 0 1 1 1 1
  spline S244 degree 3 poles (140.0927, -27.2034) (139.6235, -28.0968) (139.2283, -29.0291) (138.7712, -30.0038) knots 0 0 0 0 1 1 1 1
  spline S245 degree 3 poles (50.0849, -22.4452) (50.2926, -21.8528) (50.5007, -21.2605) (50.7079, -20.6679) knots 0 0 0 0 1 1 1 1
  spline S246 degree 3 poles (50.7079, -20.6679) (50.8123, -20.369) (50.9049, -20.0653) (51.0255, -19.7731) knots 0 0 0 0 1 1 1 1
  spline S247 degree 3 poles (51.0255, -19.7731) (51.0604, -19.6886) (51.1737, -19.5792) (51.252, -19.5784) knots 0 0 0 0 1 1 1 1
  spline S248 degree 3 poles (51.252, -19.5784) (52.4895, -19.5659) (53.7273, -19.5691) (54.965, -19.5698) knots 0 0 0 0 1 1 1 1
  spline S249 degree 3 poles (54.965, -19.5698) (55.0374, -19.5698) (55.1098, -19.5785) (55.2275, -19.5862) knots 0 0 0 0 1 1 1 1
  spline S250 degree 3 poles (55.2275, -19.5862) (54.9976, -20.2281) (54.7762, -20.8484) (54.5533, -21.4682) knots 0 0 0 0 1 1 1 1
  spline S251 degree 3 poles (54.5533, -21.4682) (52.5863, -26.939) (50.6099, -32.4064) (48.6587, -37.8828) knots 0 0 0 0 1 1 1 1
  spline S252 degree 3 poles (48.6587, -37.8828) (48.188, -39.2037) (47.7533, -40.5433) (47.5793, -41.9443) knots 0 0 0 0 1 1 1 1
  spline S253 degree 3 poles (47.5793, -41.9443) (47.5238, -42.3918) (47.5124, -42.8522) (47.5472, -43.3015) knots 0 0 0 0 1 1 1 1
  spline S254 degree 3 poles (47.5472, -43.3015) (47.5969, -43.9415) (48.0158, -44.3384) (48.6532, -44.4098) knots 0 0 0 0 1 1 1 1
  spline S255 degree 3 poles (48.6532, -44.4098) (49.495, -44.5041) (50.2819, -44.3211) (50.9682, -43.8296) knots 0 0 0 0 1 1 1 1
  spline S256 degree 3 poles (50.9682, -43.8296) (51.4214, -43.505) (51.8299, -43.117) (52.2494, -42.7473) knots 0 0 0 0 1 1 1 1
  spline S257 degree 3 poles (52.2494, -42.7473) (52.3208, -42.6843) (52.3929, -42.5673) (52.3873, -42.4803) knots 0 0 0 0 1 1 1 1
  spline S258 degree 3 poles (52.3873, -42.4803) (52.2958, -41.0495) (52.7378, -39.7205) (53.1976, -38.4066) knots 0 0 0 0 1 1 1 1
  spline S259 degree 3 poles (53.1976, -38.4066) (54.4524, -34.8214) (55.7386, -31.2473) (57.0169, -27.6704) knots 0 0 0 0 1 1 1 1
  spline S260 degree 3 poles (57.0169, -27.6704) (60.1698, -18.8474) (63.3253, -10.0253) (66.4793, -1.2026) knots 0 0 0 0 1 1 1 1
  spline S261 degree 3 poles (66.4793, -1.2026) (66.5105, -1.1153) (66.5356, -1.0258) (66.5753, -0.8998) knots 0 0 0 0 1 1 1 1
  line L22 (66.5753, -0.8998) -> (61.3495, -0.8998)
  spline S262 degree 3 poles (61.3495, -0.8998) (61.434, -0.5992) (61.5071, -0.3392) (61.5817, -0.0737) knots 0 0 0 0 1 1 1 1
  line L23 (61.5817, -0.0737) -> (70.961, -0.0737)
  spline S263 degree 3 poles (70.961, -0.0737) (70.9285, -0.1807) (70.9037, -0.2765) (70.8707, -0.3694) knots 0 0 0 0 1 1 1 1
  spline S264 degree 3 poles (70.8707, -0.3694) (66.7267, -12.0314) (62.5801, -23.6925) (58.4397, -35.3559) knots 0 0 0 0 1 1 1 1
  spline S265 degree 3 poles (58.4397, -35.3559) (57.7268, -37.364) (57.0232, -39.3758) (56.3538, -41.3985) knots 0 0 0 0 1 1 1 1
  spline S266 degree 3 poles (56.3538, -41.3985) (56.1806, -41.9219) (56.0896, -42.4913) (56.0712, -43.0432) knots 0 0 0 0 1 1 1 1
  spline S267 degree 3 poles (56.0712, -43.0432) (56.0306, -44.2662) (56.8851, -44.9938) (58.0846, -44.749) knots 0 0 0 0 1 1 1 1
  spline S268 degree 3 poles (58.0846, -44.749) (58.5682, -44.6503) (59.0639, -44.4504) (59.4731, -44.176) knots 0 0 0 0 1 1 1 1
  spline S269 degree 3 poles (59.4731, -44.176) (61.1119, -43.0774) (62.2985, -41.5649) (63.1257, -39.7979) knots 0 0 0 0 1 1 1 1
  spline S270 degree 3 poles (63.1257, -39.7979) (63.6148, -38.7533) (63.951, -37.6361) (64.3408, -36.5461) knots 0 0 0 0 1 1 1 1
  spline S271 degree 3 poles (64.3408, -36.5461) (68.5443, -24.7933) (72.7448, -13.0394) (76.9459, -1.2857) knots 0 0 0 0 1 1 1 1
  spline S272 degree 3 poles (76.9459, -1.2857) (76.9874, -1.1697) (77.0261, -1.0528) (77.0796, -0.8969) knots 0 0 0 0 1 1 1 1
  line L24 (77.0796, -0.8969) -> (71.8772, -0.8969)
  spline S273 degree 3 poles (71.8772, -0.8969) (71.8728, -0.8474) (71.8656, -0.8253) (71.87, -0.8059) knots 0 0 0 0 1 1 1 1
  spline S274 degree 2 poles (71.87, -0.8059) (72.0386, -0.0634) (72.7928, -0.0634) knots 0 0 0 1 1 1
  spline S275 degree 3 poles (72.7928, -0.0634) (75.5433, -0.0634) (78.2938, -0.0634) (81.0442, -0.0634) knots 0 0 0 0 1 1 1 1
  line L25 (81.0442, -0.0634) -> (81.4689, -0.0634)
  spline S276 degree 3 poles (81.4689, -0.0634) (81.3172, -0.5003) (81.1791, -0.9064) (81.0355, -1.3105) knots 0 0 0 0 1 1 1 1
  spline S277 degree 3 poles (81.0355, -1.3105) (76.5089, -14.0458) (71.9791, -26.78) (67.4605, -39.5181) knots 0 0 0 0 1 1 1 1
  spline S278 degree 3 poles (67.4605, -39.5181) (67.1403, -40.4209) (66.8922, -41.3499) (66.6319, -42.2727) knots 0 0 0 0 1 1 1 1
  spline S279 degree 3 poles (66.6319, -42.2727) (66.5643, -42.5124) (66.5592, -42.7745) (66.5563, -43.0267) knots 0 0 0 0 1 1 1 1
  spline S280 degree 3 poles (66.5563, -43.0267) (66.5417, -44.2641) (67.3792, -44.9721) (68.5993, -44.764) knots 0 0 0 0 1 1 1 1
  spline S281 degree 3 poles (68.5993, -44.764) (69.1748, -44.6659) (69.6796, -44.4126) (70.1463, -44.0705) knots 0 0 0 0 1 1 1 1
  spline S282 degree 3 poles (70.1463, -44.0705) (71.6905, -42.9385) (72.8455, -41.4761) (73.6418, -39.7556) knots 0 0 0 0 1 1 1 1
  spline S283 degree 3 poles (73.6418, -39.7556) (74.1085, -38.7475) (74.4293, -37.6709) (74.7999, -36.6195) knots 0 0 0 0 1 1 1 1
  spline S284 degree 3 poles (74.7999, -36.6195) (76.6624, -31.3356) (78.5196, -26.0499) (80.3787, -20.7648) knots 0 0 0 0 1 1 1 1
  spline S285 degree 3 poles (80.3787, -20.7648) (80.4133, -20.6665) (80.4479, -20.5681) (80.4962, -20.4306) knots 0 0 0 0 1 1 1 1
  line L26 (80.4962, -20.4306) -> (75.2552, -20.4306)
  spline S286 degree 3 poles (75.2552, -20.4306) (75.3359, -20.148) (75.3825, -19.9022) (75.4831, -19.6808) knots 0 0 0 0 1 1 1 1
  spline S287 degree 3 poles (75.4831, -19.6808) (75.5151, -19.6102) (75.6902, -19.574) (75.8, -19.5737) knots 0 0 0 0 1 1 1 1
  spline S288 degree 3 poles (75.8, -19.5737) (77.8099, -19.5675) (79.8199, -19.5691) (81.8299, -19.5691) knots 0 0 0 0 1 1 1 1
  spline S289 degree 3 poles (81.8299, -19.5691) (82.7185, -19.5691) (83.6071, -19.5691) (84.4957, -19.5691) knots 0 0 0 0 1 1 1 1
  line L27 (84.4957, -19.5691) -> (84.8908, -19.5691)
  spline S290 degree 3 poles (84.8908, -19.5691) (84.6969, -20.1342) (84.5194, -20.6587) (84.3372, -21.1815) knots 0 0 0 0 1 1 1 1
  spline S291 degree 3 poles (84.3372, -21.1815) (82.1946, -27.3287) (80.0448, -33.4733) (77.9153, -39.625) knots 0 0 0 0 1 1 1 1
  spline S292 degree 3 poles (77.9153, -39.625) (77.5918, -40.5594) (77.343, -41.5214) (77.099, -42.4806) knots 0 0 0 0 1 1 1 1
  spline S293 degree 3 poles (77.099, -42.4806) (77.0232, -42.7789) (77.0352, -43.1161) (77.0794, -43.4251) knots 0 0 0 0 1 1 1 1
  spline S294 degree 3 poles (77.0794, -43.4251) (77.2211, -44.4149) (78.0389, -44.9766) (79.081, -44.7494) knots 0 0 0 0 1 1 1 1
  spline S295 degree 3 poles (79.081, -44.7494) (79.5647, -44.644) (80.0606, -44.4492) (80.4698, -44.1743) knots 0 0 0 0 1 1 1 1
  spline S296 degree 3 poles (80.4698, -44.1743) (81.9568, -43.1756) (83.0471, -41.8112) (83.893, -40.2456) knots 0 0 0 0 1 1 1 1
  spline S297 degree 3 poles (83.893, -40.2456) (83.9344, -40.169) (83.9365, -40.0409) (83.9031, -39.9585) knots 0 0 0 0 1 1 1 1
  spline S298 degree 3 poles (83.9031, -39.9585) (82.6174, -36.7855) (82.7766, -33.5787) (83.9322, -30.4535) knots 0 0 0 0 1 1 1 1
  spline S299 degree 3 poles (83.9322, -30.4535) (85.9017, -25.1273) (89.5691, -21.403) (94.9427, -19.4482) knots 0 0 0 0 1 1 1 1
  spline S300 degree 3 poles (94.9427, -19.4482) (96.8678, -18.7478) (98.865, -18.5551) (100.8691, -19.0689) knots 0 0 0 0 1 1 1 1
  spline S301 degree 3 poles (100.8691, -19.0689) (103.3851, -19.714) (105.1687, -21.313) (106.3628, -23.5722) knots 0 0 0 0 1 1 1 1
  spline S302 degree 3 poles (106.3628, -23.5722) (107.5188, -25.7593) (107.8486, -28.1077) (107.5537, -30.5511) knots 0 0 0 0 1 1 1 1
  spline S303 degree 3 poles (107.5537, -30.5511) (107.0753, -34.5158) (105.1593, -37.7643) (102.4686, -40.6044) knots 0 0 0 0 1 1 1 1
  spline S304 degree 3 poles (102.4686, -40.6044) (100.6012, -42.5754) (98.3827, -44.0429) (95.8081, -44.9372) knots 0 0 0 0 1 1 1 1
  spline S305 degree 3 poles (95.8081, -44.9372) (93.5986, -45.7048) (91.3614, -45.8636) (89.1334, -45.0354) knots 0 0 0 0 1 1 1 1
  spline S306 degree 3 poles (89.1334, -45.0354) (87.2073, -44.3196) (85.7144, -43.047) (84.6127, -41.3152) knots 0 0 0 0 1 1 1 1
  spline S307 degree 3 poles (84.6127, -41.3152) (84.5617, -41.2351) (84.5132, -41.1534) (84.4605, -41.0746) knots 0 0 0 0 1 1 1 1
  spline S308 degree 3 poles (84.4605, -41.0746) (84.4504, -41.0594) (84.4258, -41.054) (84.4744, -41.0809) knots 0 0 0 0 1 1 1 1
  spline S309 degree 3 poles (84.4744, -41.0809) (83.8997, -41.8316) (83.3916, -42.6279) (82.7546, -43.3024) knots 0 0 0 0 1 1 1 1
  spline S310 degree 3 poles (82.7546, -43.3024) (80.844, -45.3252) (78.4925, -45.9992) (75.7898, -45.3455) knots 0 0 0 0 1 1 1 1
  spline S311 degree 3 poles (75.7898, -45.3455) (74.2035, -44.9618) (73.427, -43.9443) (73.377, -42.3173) knots 0 0 0 0 1 1 1 1
  spline S312 degree 3 poles (73.377, -42.3173) (73.3743, -42.2262) (73.3767, -42.1348) (73.3767, -41.9795) knots 0 0 0 0 1 1 1 1
  spline S313 degree 3 poles (73.3767, -41.9795) (73.0458, -42.3875) (72.7758, -42.7603) (72.4656, -43.096) knots 0 0 0 0 1 1 1 1
  spline S314 degree 3 poles (72.4656, -43.096) (71.2784, -44.3806) (69.8832, -45.31) (68.0996, -45.5148) knots 0 0 0 0 1 1 1 1
  spline S315 degree 3 poles (68.0996, -45.5148) (67.0306, -45.6375) (65.9669, -45.6042) (64.9382, -45.2356) knots 0 0 0 0 1 1 1 1
  spline S316 degree 3 poles (64.9382, -45.2356) (63.5857, -44.7511) (62.923, -43.8262) (62.8928, -42.3877) knots 0 0 0 0 1 1 1 1
  spline S317 degree 3 poles (62.8928, -42.3877) (62.8902, -42.2662) (62.8925, -42.1445) (62.8925, -41.9728) knots 0 0 0 0 1 1 1 1
  spline S318 degree 3 poles (62.8925, -41.9728) (62.5336, -42.4076) (62.2327, -42.813) (61.8902, -43.1798) knots 0 0 0 0 1 1 1 1
  spline S319 degree 3 poles (61.8902, -43.1798) (60.4964, -44.6726) (58.821, -45.5971) (56.731, -45.5649) knots 0 0 0 0 1 1 1 1
  spline S320 degree 3 poles (56.731, -45.5649) (56.0409, -45.5543) (55.3375, -45.4608) (54.6679, -45.2941) knots 0 0 0 0 1 1 1 1
  spline S321 degree 3 poles (54.6679, -45.2941) (53.5786, -45.0228) (53.0763, -44.5495) (52.6072, -43.5745) knots 0 0 0 0 1 1 1 1
  spline S322 degree 3 poles (52.6072, -43.5745) (52.0194, -43.9749) (51.4482, -44.4101) (50.8342, -44.773) knots 0 0 0 0 1 1 1 1
  spline S323 degree 3 poles (50.8342, -44.773) (49.3654, -45.6409) (47.775, -45.7703) (46.1469, -45.3786) knots 0 0 0 0 1 1 1 1
  spline S324 degree 3 poles (46.1469, -45.3786) (44.7538, -45.0434) (43.9596, -44.0239) (43.8607, -42.5731) knots 0 0 0 0 1 1 1 1
  spline S325 degree 3 poles (43.8607, -42.5731) (43.7805, -41.3953) (44.0412, -40.2656) (44.3478, -39.1425) knots 0 0 0 0 1 1 1 1
  spline S326 degree 3 poles (44.3478, -39.1425) (44.3802, -39.0239) (44.4122, -38.9052) (44.3822, -38.747) knots 0 0 0 0 1 1 1 1
  spline S327 degree 3 poles (44.3822, -38.747) (44.2975, -38.8447) (44.2114, -38.9412) (44.1283, -39.0402) knots 0 0 0 0 1 1 1 1
  spline S328 degree 3 poles (44.1283, -39.0402) (42.8844, -40.5225) (41.6555, -42.0196) (40.0946, -43.1941) knots 0 0 0 0 1 1 1 1
  spline S329 degree 3 poles (40.0946, -43.1941) (38.6342, -44.293) (37.0632, -45.1607) (35.2298, -45.4504) knots 0 0 0 0 1 1 1 1
  spline S330 degree 3 poles (35.2298, -45.4504) (33.7641, -45.6821) (32.3176, -45.6378) (30.9433, -45.0022) knots 0 0 0 0 1 1 1 1
  spline S331 degree 3 poles (30.9433, -45.0022) (29.1176, -44.1579) (28.0823, -42.6659) (27.6348, -40.7633) knots 0 0 0 0 1 1 1 1
  spline S332 degree 3 poles (27.6348, -40.7633) (27.443, -39.948) (27.4212, -39.0926) (27.3272, -38.2549) knots 0 0 0 0 1 1 1 1
  spline S333 degree 3 poles (27.3272, -38.2549) (27.3127, -38.1253) (27.3252, -37.9926) (27.2528, -37.8437) knots 0 0 0 0 1 1 1 1
  spline S334 degree 3 poles (27.2528, -37.8437) (27.118, -38.0638) (26.9879, -38.287) (26.8476, -38.5034) knots 0 0 0 0 1 1 1 1
  spline S335 degree 3 poles (26.8476, -38.5034) (24.8612, -41.5667) (22.1611, -43.7524) (18.7272, -44.9928) knots 0 0 0 0 1 1 1 1
  spline S336 degree 3 poles (18.7272, -44.9928) (16.8655, -45.6654) (14.9147, -45.7043) (12.9615, -45.5794) knots 0 0 0 0 1 1 1 1
  spline S337 degree 3 poles (12.9615, -45.5794) (11.4556, -45.483) (9.982, -45.2081) (8.5868, -44.6156) knots 0 0 0 0 1 1 1 1
  spline S338 degree 3 poles (8.5868, -44.6156) (5.0699, -43.1219) (2.7269, -40.5128) (1.4018, -36.9651) knots 0 0 0 0 1 1 1 1
  spline S339 degree 3 poles (1.4018, -36.9651) (0.5889, -34.789) (0.2461, -32.5189) (0.1152, -30.2088) knots 0 0 0 0 1 1 1 1
  spline S340 degree 3 poles (0.1152, -30.2088) (-0.1988, -24.667) (1.4603, -19.6798) (4.4487, -15.0988) knots 0 0 0 0 1 1 1 1
  spline S341 degree 3 poles (4.4487, -15.0988) (7.6391, -10.2081) (11.8716, -6.4708) (17.171, -3.9759) knots 0 0 0 0 1 1 1 1
  spline S342 degree 3 poles (17.171, -3.9759) (18.9174, -3.1537) (20.7361, -2.5457) (22.6573, -2.2749) knots 0 0 0 0 1 1 1 1
  spline S343 degree 3 poles (22.6573, -2.2749) (25.2538, -1.9088) (27.7778, -2.2096) (30.2365, -3.0973) knots 0 0 0 0 1 1 1 1
  spline S344 degree 3 poles (30.2365, -3.0973) (31.1101, -3.4127) (31.9675, -3.7753) (32.8488, -4.0666) knots 0 0 0 0 1 1 1 1
  spline S345 degree 3 poles (32.8488, -4.0666) (33.3657, -4.2376) (33.9099, -4.3637) (34.4509, -4.4166) knots 0 0 0 0 1 1 1 1
  spline S346 degree 3 poles (34.4509, -4.4166) (35.5622, -4.5251) (36.3629, -3.9783) (36.9084, -3.0554) knots 0 0 0 0 1 1 1 1
  spline S347 degree 3 poles (36.9084, -3.0554) (37.0752, -2.7732) (37.2322, -2.6868) (37.5281, -2.7909) knots 0 0 0 0 1 1 1 1
  spline S348 degree 3 poles (37.5281, -2.7909) (37.6735, -2.8421) (37.8301, -2.8615) (38.014, -2.9026) knots 0 0 0 0 1 1 1 1
  spline S349 degree 3 poles (38.014, -2.9026) (37.7215, -3.721) (37.4387, -4.513) (37.1555, -5.3048) knots 0 0 0 0 1 1 1 1
  spline S350 degree 3 poles (37.1555, -5.3048) (36.1535, -8.1065) (35.1509, -10.908) (34.1497, -13.71) knots 0 0 0 0 1 1 1 1
  spline S351 degree 3 poles (34.1497, -13.71) (33.9218, -14.3478) (33.924, -14.3486) (33.1894, -14.2539) knots 0 0 0 0 1 1 1 1
  spline S352 degree 3 poles (33.1894, -14.2539) (33.2661, -13.6185) (33.3592, -12.9843) (33.4161, -12.3467) knots 0 0 0 0 1 1 1 1
  spline S353 degree 3 poles (33.4161, -12.3467) (33.5354, -11.0084) (33.6343, -9.6642) (33.2979, -8.3429) knots 0 0 0 0 1 1 1 1
  spline S354 degree 3 poles (33.2979, -8.3429) (32.7503, -6.1919) (31.4072, -4.6744) (29.3636, -3.8873) knots 0 0 0 0 1 1 1 1
  spline S355 degree 3 poles (29.3636, -3.8873) (25.4024, -2.3618) (21.6115, -2.5974) (18.1064, -5.2075) knots 0 0 0 0 1 1 1 1
  spline S356 degree 3 poles (18.1064, -5.2075) (15.5983, -7.0752) (13.6497, -9.4342) (12.0128, -12.064) knots 0 0 0 0 1 1 1 1
  spline S357 degree 3 poles (12.0128, -12.064) (9.4965, -16.1067) (7.7161, -20.4766) (6.3534, -25.0241) knots 0 0 0 0 1 1 1 1
  spline S358 degree 3 poles (6.3534, -25.0241) (5.5761, -27.6183) (5.0135, -30.2599) (4.7229, -32.9543) knots 0 0 0 0 1 1 1 1
  spline S359 degree 3 poles (4.7229, -32.9543) (4.5192, -34.842) (4.4781, -36.7259) (4.9304, -38.5933) knots 0 0 0 0 1 1 1 1
  spline S360 degree 3 poles (4.9304, -38.5933) (5.6053, -41.3794) (7.3021, -43.2695) (10.0108, -44.1478) knots 0 0 0 0 1 1 1 1
  spline S361 degree 3 poles (10.0108, -44.1478) (13.1649, -45.1705) (16.3359, -45.2186) (19.4152, -43.8207) knots 0 0 0 0 1 1 1 1
  spline S362 degree 3 poles (19.4152, -43.8207) (22.1935, -42.5594) (24.3784, -40.5957) (26.0144, -38.024) knots 0 0 0 0 1 1 1 1
  spline S363 degree 3 poles (26.0144, -38.024) (26.4452, -37.3469) (26.7981, -36.6105) (27.2978, -35.9909) knots 0 0 0 0 1 1 1 1
  spline S364 degree 3 poles (27.2978, -35.9909) (27.6013, -35.6146) (27.6548, -35.2071) (27.7761, -34.8009) knots 0 0 0 0 1 1 1 1
  spline S365 degree 3 poles (27.7761, -34.8009) (28.5607, -32.172) (29.8681, -29.8167) (31.5841, -27.6967) knots 0 0 0 0 1 1 1 1
  spline S366 degree 3 poles (31.5841, -27.6967) (34.2471, -24.4068) (37.4617, -21.785) (41.2974, -19.9603) knots 0 0 0 0 1 1 1 1